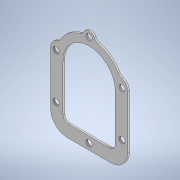
# Autodesk Inventor part: 74. Крышка люка
Saved by Autodesk Inventor 2021 (Build 250183000, 183)
## iProperties
Created: 2021-03-11
Part Number: 74. Крышка люка
Material: Типовые
Document SubType Name: Modeling
Designer: Данил
Density: 1 g/cm^3
Appearance: По умолчанию
Author: Данил
Autodesk Inventor part; units mm, degrees
ref_plane "YZ Plane" through (0, 0, 0) normal (1, 0, 0) x (0, 1, 0)
ref_plane "XZ Plane" through (0, 0, 0) normal (0, 1, 0) x (-1, 0, 0)
ref_plane "XY Plane" through (0, 0, 0) normal (0, 0, 1) x (1, 0, 0)
sketch "Эскиз1" plane through (0, 0, 0) normal (0, 0, 1) x (1, 0, 0)
  line L0 (0, 91.5) -> (0, -91.5) construction
  line L1 (-68.5, 0) -> (68.5, 0) construction
  circle A0 centre (0, -80.5) radius 5.4
  line L2 (-38.5, -91.5) -> (38.5, -91.5)
  line L3 (-68.5, -61.5) -> (-68.5, 33.5)
  line L4 (68.5, -61.5) -> (68.5, 33.5)
  arc A1 (-68.5, -61.5) -> (-38.5, -91.5) centre (-38.5, -61.5) ccw
  arc A2 (38.5, -91.5) -> (68.5, -61.5) centre (38.5, -61.5) ccw
  line L5 (-36.5, -69.5) -> (36.5, -69.5)
  line L6 (-46.5, -59.5) -> (-46.5, 22.5)
  line L7 (46.5, -59.5) -> (46.5, 22.5)
  arc A3 (-46.5, -59.5) -> (-36.5, -69.5) centre (-36.5, -59.5) ccw
  arc A4 (36.5, -69.5) -> (46.5, -59.5) centre (36.5, -59.5) ccw
  arc A5 (-57.7881, 47.874) -> (-68.5, 33.5) centre (-53.5, 33.5) ccw
  arc A6 (-57.7881, 47.874) -> (-51.9829, 52.4629) centre (-60.6468, 57.4567) ccw
  arc A7 (-15.8919, 80.3571) -> (-51.9829, 52.4629) centre (0, 22.5) ccw
  arc A8 (-15.8919, 80.3571) -> (-9.2702, 86.25) centre (-18.5405, 90) ccw
  arc A9 (9.2702, 86.25) -> (-9.2702, 86.25) centre (0, 82.5) ccw
  arc A10 (9.2702, 86.25) -> (15.8919, 80.3571) centre (18.5405, 90) ccw
  arc A11 (51.9829, 52.4629) -> (15.8919, 80.3571) centre (0, 22.5) ccw
  arc A12 (51.9829, 52.4629) -> (57.7881, 47.874) centre (60.6468, 57.4567) ccw
  arc A13 (68.5, 33.5) -> (57.7881, 47.874) centre (53.5, 33.5) ccw
  circle A14 centre (0, 82.5) radius 5.4
  circle A15 centre (-58.5, 33.5) radius 5.4
  circle A16 centre (58.5, 33.5) radius 5.4
  circle A17 centre (-58.5, -46.5) radius 5.4
  circle A18 centre (58.5, -46.5) radius 5.4
  arc A19 (46.5, 22.5) -> (-46.5, 22.5) centre (0, 22.5) ccw
  point P0 (0, 0)
  point P1 (0, 0)
  point P2 (0, 0)
  point P3 (-68.5, -91.5)
  point P4 (68.5, -91.5)
  point P5 (0, -91.5)
  point P6 (-46.5, -69.5)
  point P7 (46.5, -69.5)
  point P8 (0, -69.5)
  point P9 (0, -6.5)
  dimension "d2" = 183
  dimension "d3" = 137
  dimension "d4" = 10.8
  dimension "d5" = 30
  dimension "d6" = 93
  dimension "d7" = 22
  dimension "d8" = 11
  dimension "d9" = 10
  dimension "d10" = 15
  dimension "d11" = 10
  dimension "d12" = 103
  dimension "d13" = 60
  dimension "d14" = 10
  dimension "d15" = 10
  dimension "d16" = 163
  dimension "d17" = 114
  dimension "d18" = 10
  dimension "d19" = 60
  dimension "d20" = 10
  dimension "d21" = 15
  dimension "d22" = 74
  dimension "d23" = 10.8
  dimension "d24" = 12
  dimension "d25" = 40
  dimension "d26" = 12
  dimension "d29" = 80
  constraints: 28 point on circle, 20 centre point, 20 tangent, 16 end point, 12 point on line, 7 coincident, 6 vertical, 4 equal radius, 4 midpoint, 3 horizontal, 3 vertical alignment, 2 horizontal alignment, 4 other
  measures "d2" distance of L0.start L0.end
  measures "d3" distance of L1.start L1.end
  measures "d4" diameter of A0
  measures "d5" radius of A1
  measures "d6" distance of point (-46.5, -69.5) point (46.5, -69.5)
  measures "d7" distance between parallel lines of L2 L5
  measures "d8" distance from line of L5 A0.centre
  measures "d9" radius of A3
  measures "d10" radius of A5
  measures "d11" radius of A6
  measures "d12" distance of A0.centre point (0, 22.5)
  measures "d13" radius of A7
  measures "d14" radius of A8
  measures "d15" radius of A9
  measures "d16" distance of A0.centre A9.centre
  measures "d17" vertical distance of A0.centre A5.centre
  measures "d18" radius of A10
  measures "d19" radius of A11
  measures "d20" radius of A12
  measures "d21" radius of A13
  measures "d22" distance of A0.centre point (0, -6.5)
  measures "d23" diameter of A14
  measures "d24" distance from line of L6 A15.centre
  measures "d25" vertical distance of point (0, -6.5) A15.centre
  measures "d26" distance from line of L7 A16.centre
  measures "d29" distance of A15.centre A17.centre
extrude "Выдавливание1" add sketch "Эскиз1" along normal blind 3
